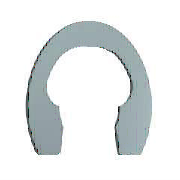
# Autodesk Inventor part: ASME B27.8M - 3EM1-11
Saved by Autodesk Inventor 2022 (Build 260153000, 153)
## iProperties
Created: 2021-02-02
Part Number: ASME B27.8M - 3EM1-11
Material: 钢，软
Description: 通用公制锥形和异径横截面挡圈 - 类型 3EM1
Document SubType Name: Modeling
Standard: ASME B27.8M
Designer: Lzy18
Standard Revision: 1999
Standards Organization: ANSI
Language: zh-CN
Size Designation: 3EM1-11
Categories: <MemberInstance><Categories><Category DisplayName="轴用零件" InternalName="7f7aeb1f-a693-4053-b835-cee3144e0d98" Mnemonic="SHFT"><Category DisplayName="弹性挡圈" InternalName="413b042a-1f46-4051-a560-0e0e417af91f" Mnemonic="CLIP"><CategoryParameter DisplayName="厚度" InternalName="230c7f7c-2544-4c6d-b8d5-773e831b23fa" Mnemonic="thick"/><CategoryParameter DisplayName="沟槽直径" InternalName="4054b45c-161d-4ad6-befb-f30b3855ce84" Mnemonic="grvdia"/><CategoryParameter DisplayName="沟槽宽度" InternalName="4dde6996-4bf1-443b-8317-d4f4fc6b9be0" Mnemonic="NB"/><CategoryParameter DisplayName="轴直径" InternalName="a433c9ab-b9eb-4798-a453-f2210a67728e" Mnemonic="shaftdia"/><Category DisplayName="轴用弹性挡圈" InternalName="a9a2b132-a8be-48ab-9c3d-0c324a909558" Mnemonic="OUCLIP"><CategoryParameter DisplayName="最小轴直径" InternalName="62b77b9b-1e86-4b9a-9911-d7c0fa48fc9a" Mnemonic="shaftdiamin"/><CategoryParameter DisplayName="外径" InternalName="a3599e7b-be7c-41b5-9a50-6dab253b0906" Mnemonic="outdia"/></Category></Category></Category><Category DisplayName="数据类型" InternalName="23b78d0f-2648-40c6-8793-ca6db495c9e8" Mnemonic="DATATYPE"><CategoryParameter DisplayName="显示名" InternalName="05415f3d-3907-474b-a020-eb9d644f4cf3" Mnemonic="DISPLAYNAME"/><CategoryParameter DisplayName="标准" InternalName="0c0a119c-1e12-4c84-803f-101930972f5e" Mnemonic="STANDARD"/><CategoryParameter DisplayName="描述" InternalName="13903e3d-64b1-4950-80da-f627842ea37f" Mnemonic="DESCRIPTION"/><CategoryParameter DisplayName="规格" InternalName="2675968c-4ce5-49e0-a4f5-552d29089031" Mnemonic="DESIGNATION"/><CategoryParameter DisplayName="默认列" InternalName="2af9ec52-faaa-4026-b378-f9fa4afca842" Mnemonic="DEFAULTROW"/><CategoryParameter DisplayName="文件夹名称" InternalName="3f06958e-8713-4116-9be7-ed6184ecc97b" Mnemonic="FOLDERNAME"/><CategoryParameter DisplayName="版本指南" InternalName="45a75005-10b1-4dfc-8d6d-dfe629f0b93c" Mnemonic="REVISIONGUID"/><CategoryParameter DisplayName="文件名" InternalName="8b46a4cc-9585-4fed-90c3-899f57e09a73" Mnemonic="FILENAME"/><CategoryParameter DisplayName="标准组织" InternalName="8f5914e1-4693-403f-8ab5-d37768198c9d" Mnemonic="STDSORG"/><CategoryParameter DisplayName="系列版本" InternalName="914462f6-6e19-4b14-ba84-155b9680b1d0" Mnemonic="FAMILYREVISION"/><CategoryParameter DisplayName="标准版本" InternalName="91d5a463-65c2-4fde-b823-3b7fea5e8e17" Mnemonic="STANDARDREVISION"/><CategoryParameter DisplayName="成员版本" InternalName="a65d44b9-392f-4f4f-857b-e4b3d54996fe" Mnemonic="MEMBERREVISION"/><CategoryParameter DisplayName="剪裁格式" InternalName="bc51e27b-3422-4e78-93ef-cec197ddf230" Mnemonic="CLIPFORMAT"/><CategoryParameter DisplayName="制造商" InternalName="cd6c7a72-a28a-4e50-99a9-2c7f4e13e5ad" Mnemonic="MANUFACTURER"/><CategoryParameter DisplayName="内部名称" InternalName="cf1d0246-76d9-4b4a-8305-fa0409afb5c1" Mnemonic="INTERNALNAME"/><CategoryParameter DisplayName="是否公制" InternalName="e2385c5b-1ea4-4823-96a8-8de651266ec3" Mnemonic="ISMETRIC"/><Category DisplayName="零件" InternalName="c0e0b642-3bcb-4cc8-9e80-f96d35c4afa4" Mnemonic="PART"><CategoryParameter DisplayName="零件代号" InternalName="016b6077-bfbe-49bd-92c9-d8d59c39c941" Mnemonic="PARTNUMBER"/><CategoryParameter DisplayName="库存编号" InternalName="4dba7c1c-e26c-444e-836c-b08b433409a8" Mnemonic="STOCKNUMBER"/><CategoryParameter DisplayName="材料键" InternalName="5c9a8adb-dd2b-4535-b97f-0a94a95fe41f" Mnemonic="MATERIALKEY"/><CategoryParameter DisplayName="材料" InternalName="818a152a-d3c3-49ca-80ee-df7d91421b8e" Mnemonic="MATERIAL"/></Category></Category><Category DisplayName="先前版本映射 DA" InternalName="924fff40-ddd0-4eff-ad42-30e3774ef79e" Mnemonic="LEGACYMAPDA"><CategoryParameter DisplayName="DACookie" InternalName="316934ee-8fe1-4c7a-9c36-f2d79e1add1a" Mnemonic="DACOOKIE"/></Category></Categories><FamilyTemplate Id="AB278Me"><FamilyTemplateParameters><FamilyTemplateParameter ObjectType="kUserParameterObject" ValueType="xs:double" Id="1" ObjectReferenceKey="sd"/><FamilyTemplateParameter ObjectType="kUserParameterObject" ValueType="xs:double" Id="2" ObjectReferenceKey="Diam2"/><FamilyTemplateParameter ObjectType="kUserParameterObject" ValueType="xs:double" Id="5" ObjectReferenceKey="t1"/><FamilyTemplateParameter ObjectType="kUserParameterObject" ValueType="xs:double" Id="8" ObjectReferenceKey="l2"/><FamilyTemplateParameter ObjectType="kUserParameterObject" ValueType="xs:string" Id="117" ObjectReferenceKey="TEMPLATE"/><FamilyTemplateParameter ObjectType="kPropertyObject" ValueType="xs:string" Id="100" ObjectReferenceKey="{32853F0F-3444-11d1-9E93-0060B03C1CA6}" SubObjectId="52"/><FamilyTemplateParameter ObjectType="kPropertyObject" ValueType="xs:string" Id="105" ObjectReferenceKey="{32853F0F-3444-11d1-9E93-0060B03C1CA6}" SubObjectId="5"/><FamilyTemplateParameter ObjectType="kPartComponentDefinitionObject" ValueType="xs:string" Id="110" SubObjectId="Material"/></FamilyTemplateParameters></FamilyTemplate><CategoryParameterMap><ParamToTemplateMap><ParamToTemplate CategoryParameter="//CategoryParameter[@InternalName='05415f3d-3907-474b-a020-eb9d644f4cf3']" ConstantValue="ASME B27.8M"/><ParamToTemplate CategoryParameter="//CategoryParameter[@InternalName='cf1d0246-76d9-4b4a-8305-fa0409afb5c1']" ConstantValue="D52488CB-E0F0-414B-9693-66AA36E87DF7"/><ParamToTemplate CategoryParameter="//CategoryParameter[@InternalName='3f06958e-8713-4116-9be7-ed6184ecc97b']" ConstantValue="ASME B27.8M(2)"/><ParamToTemplate CategoryParameter="//CategoryParameter[@InternalName='914462f6-6e19-4b14-ba84-155b9680b1d0']" ConstantValue="10"/><ParamToTemplate CategoryParameter="//CategoryParameter[@InternalName='bc51e27b-3422-4e78-93ef-cec197ddf230']" ConstantValue="CF_INVENTOR.STDPARTS"/><ParamToTemplate CategoryParameter="//CategoryParameter[@InternalName='e2385c5b-1ea4-4823-96a8-8de651266ec3']" ConstantValue="true"/><ParamToTemplate CategoryParameter="//CategoryParameter[@InternalName='13903e3d-64b1-4950-80da-f627842ea37f']" ConstantValue="General Purpose Metric Tapered and Reduced Cross Section Retaining Ring -Type 3EM1"/><ParamToTemplate CategoryParameter="//CategoryParameter[@InternalName='8f5914e1-4693-403f-8ab5-d37768198c9d']" ConstantValue="ANSI"/><ParamToTemplate CategoryParameter="//CategoryParameter[@InternalName='0c0a119c-1e12-4c84-803f-101930972f5e']" ConstantValue="ASME B27.8M"/><ParamToTemplate CategoryParameter="//CategoryParameter[@InternalName='cd6c7a72-a28a-4e50-99a9-2c7f4e13e5ad']" TemplateParameter="104"/><ParamToTemplate CategoryParameter="//CategoryParameter[@InternalName='91d5a463-65c2-4fde-b823-3b7fea5e8e17']" ConstantValue="1999"/><ParamToTemplate CategoryParameter="//CategoryParameter[@InternalName='45a75005-10b1-4dfc-8d6d-dfe629f0b93c']" ConstantValue="3f8fe9f5-c015-42f6-a75b-ce2af8096aa6"/><ParamToTemplate CategoryParameter="//CategoryParameter[@InternalName='2af9ec52-faaa-4026-b378-f9fa4afca842']" ConstantValue="10"/><ParamToTemplate CategoryParameter="//CategoryParameter[@InternalName='8b46a4cc-9585-4fed-90c3-899f57e09a73']" ConstantValue="ASME B27.8M - 3EM1-11"/><ParamToTemplate CategoryParameter="//CategoryParameter[@InternalName='a65d44b9-392f-4f4f-857b-e4b3d54996fe']" ConstantValue="5A120D9C-9A6A-4CBD-889F-96B5626AA826"/><ParamToTemplate CategoryParameter="//CategoryParameter[@InternalName='4dde6996-4bf1-443b-8317-d4f4fc6b9be0']" ConstantValue="1"/><ParamToTemplate CategoryParameter="//CategoryParameter[@InternalName='316934ee-8fe1-4c7a-9c36-f2d79e1add1a']" ConstantValue="*ANS~AB278ME~3EM1-11*"/><ParamToTemplate CategoryParameter="//CategoryParameter[@InternalName='2675968c-4ce5-49e0-a4f5-552d29089031']" TemplateParameter="100"/><ParamToTemplate CategoryParameter="//CategoryParameter[@InternalName='4054b45c-161d-4ad6-befb-f30b3855ce84']" TemplateParameter="2"/><ParamToTemplate CategoryParameter="//CategoryParameter[@InternalName='818a152a-d3c3-49ca-80ee-df7d91421b8e']" TemplateParameter="110"/><ParamToTemplate CategoryParameter="//CategoryParameter[@InternalName='016b6077-bfbe-49bd-92c9-d8d59c39c941']" TemplateParameter="105"/><ParamToTemplate CategoryParameter="//CategoryParameter[@InternalName='a433c9ab-b9eb-4798-a453-f2210a67728e']" TemplateParameter="1"/><ParamToTemplate CategoryParameter="//CategoryParameter[@InternalName='230c7f7c-2544-4c6d-b8d5-773e831b23fa']" TemplateParameter="5"/></ParamToTemplateMap></CategoryParameterMap></MemberInstance>
Density: 7.85 g/cm^3
Appearance: 半抛光
IsCustomPart: 0
Author: Lzy18
Autodesk Inventor part; units mm, degrees
ref_plane "YZ Plane" through (0, 0, 0) normal (1, 0, 0) x (0, 1, 0)
ref_plane "XZ Plane" through (0, 0, 0) normal (0, 1, 0) x (-1, 0, 0)
ref_plane "XY Plane" through (0, 0, 0) normal (0, 0, 1) x (1, 0, 0)
sketch "草图2" plane through (0, 0, 0) normal (0, 0, 1) x (1, 0, 0)
  line L0 (-6.9375, 0) -> (-4.4, 0)
  arc A0 (-0.9227, 6.8759) -> (-6.9375, 0) centre (0, 0) ccw
  line L1 (-0.9227, 6.8759) -> (-0.9227, 4.3022)
  arc A1 (0.9227, 4.3022) -> (-0.9227, 4.3022) centre (0, 0) ccw
  line L2 (0.9227, 4.3022) -> (0.9227, 6.8759)
  arc A2 (6.9375, 0) -> (0.9227, 6.8759) centre (0, 0) ccw
  line L3 (4.4, 0) -> (6.9375, 0)
  arc A3 (6.7982, -6.6) -> (-6.7982, -6.6) centre (0, 0) ccw
  line L4 (0, -3.55) -> (0, 5.55) projected
  line L5 (-4.4, 0) -> (-4.4, -6.6)
  line L6 (-4.4, -6.6) -> (-6.7982, -6.6)
  line L7 (4.4, 0) -> (4.4, -6.6)
  line L8 (4.4, -6.6) -> (6.7982, -6.6)
  dimension "d29" = 18.95
  dimension "d33" = 13.875
  dimension "d39" = 0.9227
  dimension "d40" = 4.4
  dimension "d41" = 6.6
  constraints: 16 end point, 10 point on circle, 5 horizontal alignment, 4 centre point, 3 coincident, 2 horizontal, 2 perpendicular, 2 point on line, 2 vertical, 1 collinear, 1 concentric, 1 parallel
  measures "d29" diameter of A3
  measures "d33" diameter of A0
  measures "d39" distance between parallel lines of L4 L1
  measures "d40" radius of A1
  measures "d41" distance from line of A1.centre L6
extrude "拉伸1" add sketch "草图2" along normal blind 0.9
fillet "圆角1" radius 1.2687 4 edges at (-6.9375, 0, 0.45) (-0.9227, 6.8759, 0.45) (0.9227, 6.8759, 0.45) (6.9375, 0, 0.45)
fillet "圆角2" radius 2.9333 2 edges at (-4.4, -6.6, 0.45) (4.4, -6.6, 0.45)
equation "\"d29\" = l2"
equation "\"d33\" = 0.5 * Diam2 + 0.5 * l2"
equation "\"d39\" = -0.0909091 * Diam2 + 0.0909091 * l2"
equation "\"d40\" = 0.5 * Diam2"
equation "\"d41\" = 0.75 * Diam2"
equation "\"d20\" = t1"
equation "\"d22\" = -0.125 * Diam2 + 0.125 * l2"
equation "\"d42\" = 0.333333 * Diam2"
equation "\"l2\" = 18.95"
equation "\"t1\" = 0.9"
equation "\"Diam2\" = 8.8"
equation "\"sd\" = 11"
equation "\"TEMPLATE\" = 1.2345"
body "Solid1"
